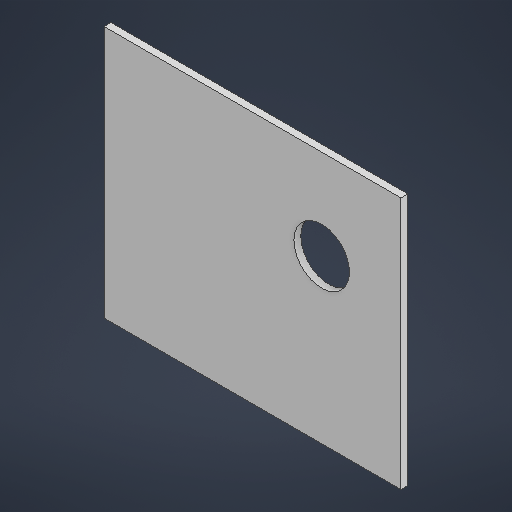
# Autodesk Inventor part: tapa_arriba
Saved by Autodesk Inventor 2026.2 (Build 302298010, 298A)
## iProperties
Created: 2026-03-16
Part Number: tapa_arriba
Material: Generic
Document SubType Name: Modeling
Designer: trini
Density: 1 g/cm^3
Appearance: Default
Author: trini
Autodesk Inventor part; units mm, degrees
ref_plane "YZ Plane" through (0, 0, 0) normal (1, 0, 0) x (0, 1, 0)
ref_plane "XZ Plane" through (0, 0, 0) normal (0, 1, 0) x (-1, 0, 0)
ref_plane "XY Plane" through (0, 0, 0) normal (0, 0, 1) x (1, 0, 0)
sketch "Sketch1" plane through (0, 0, 0) normal (0, 0, 1) x (1, 0, 0)
  line L0 (-107, -91) -> (107, -91)
  line L1 (107, -91) -> (107, 91)
  line L2 (107, 91) -> (-107, 91)
  line L3 (-107, 91) -> (-107, -91)
  line L4 (-107, -91) -> (107, 91) construction
  line L5 (107, -91) -> (-107, 91) construction
  point P0 (0, 0)
  dimension "d0" = 214
  dimension "d1" = 182
  constraints: 12 end point, 2 midpoint, 2 parallel, 1 horizontal, 1 perpendicular
  measures "d0" distance of L1.end L2.end
  measures "d1" distance of L0.end L1.end
extrude "Extrusion1" add sketch "Sketch1" along normal blind 5
sketch "Sketch2" plane through (0, 0, 0) normal (0, 0, -1) x (-1, 0, 0)
  circle A0 centre (-49.8, 26.07) radius 20
  line L0 (-107, -91) -> (-107, 91) projected
  line L1 (107, -91) -> (-107, -91) projected
  point P0 (0, 0)
  dimension "d4" = 57.2
  dimension "d5" = 40
  dimension "d6" = 117.07
  constraints: 1 centre point
  measures "d4" distance from line of L0 A0.centre
  measures "d5" diameter of A0
  measures "d6" distance from line of L1 A0.centre
extrude "Extrusion2" cut sketch "Sketch2" against normal blind 5
body "Solid1"
